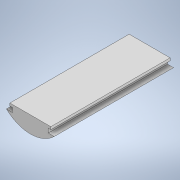
# Autodesk Inventor part: cap
Saved by Autodesk Inventor 2020 (Build 240168000, 168)
## iProperties
Created: 2022-10-17
Part Number: cap
Material: Типовые
Document SubType Name: Modeling
Designer: zigma
Density: 1 g/cm^3
Appearance: По умолчанию
Author: zigma
Autodesk Inventor part; units mm, degrees
ref_plane "YZ Plane" through (0, 0, 0) normal (1, 0, 0) x (0, 1, 0)
ref_plane "XZ Plane" through (0, 0, 0) normal (0, 1, 0) x (-1, 0, 0)
ref_plane "XY Plane" through (0, 0, 0) normal (0, 0, 1) x (1, 0, 0)
sketch "Эскиз1" plane through (0, 0, 0) normal (0, 0, 1) x (1, 0, 0)
  arc A0 (-14.0253, -14.258) -> (14.0253, -14.258) centre (0, 0) ccw
  line L0 (0, 0) -> (0, -20) construction
  line L1 (-10.5193, -14.258) -> (-10.5193, -11.758)
  line L2 (-10.5193, -11.758) -> (-12.0193, -11.758)
  line L3 (-12.0193, -11.758) -> (-12.0193, -10.258)
  line L4 (-12.0193, -10.258) -> (0, -10.258)
  line L5 (10.5193, -14.258) -> (10.5193, -11.758)
  line L6 (10.5193, -11.758) -> (12.0193, -11.758)
  line L7 (12.0193, -11.758) -> (12.0193, -10.258)
  line L8 (12.0193, -10.258) -> (0, -10.258)
  line L9 (-14.0253, -14.258) -> (-10.5193, -14.258)
  line L10 (10.5193, -14.258) -> (14.0253, -14.258)
  dimension "d0" = 40
  dimension "d2" = 2.5
  dimension "d3" = 1.5
  dimension "d4" = 1.5
  dimension "d5" = 3.506
  constraints: 22 end point, 4 symmetric about line, 3 perpendicular, 3 point on circle, 2 horizontal, 2 vertical, 1 centre point, 1 coincident, 1 point on line
  measures "d0" diameter of A0
  measures "d2" distance of L1.start L1.end
  measures "d3" distance of L1.end L2.end
  measures "d4" distance of L2.end L3.end
  measures "d5" distance from line of L9.start L1
extrude "Выдавливание1" add sketch "Эскиз1" along normal blind 70
